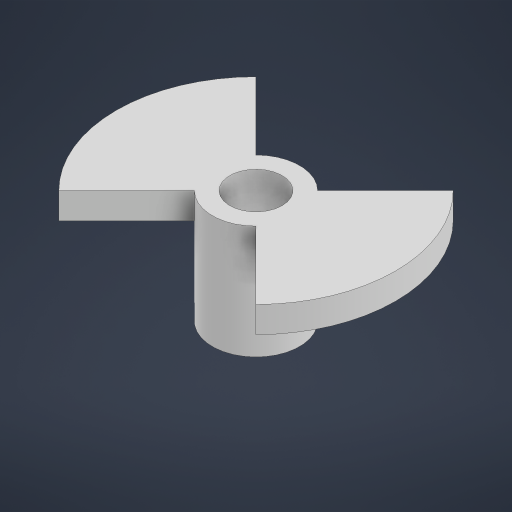
# Autodesk Inventor part: Helice
Saved by Autodesk Inventor 2023.4 (Build 274418000, 418)
## iProperties
Created: 2024-07-01
Part Number: Helice
Material: Generic
Document SubType Name: Modeling
Designer: danni
Density: 1 g/cm^3
Appearance: Default
Author: danni
Autodesk Inventor part; units mm, degrees
ref_plane "YZ Plane" through (0, 0, 0) normal (1, 0, 0) x (0, 1, 0)
ref_plane "XZ Plane" through (0, 0, 0) normal (0, 1, 0) x (-1, 0, 0)
ref_plane "XY Plane" through (0, 0, 0) normal (0, 0, 1) x (1, 0, 0)
sketch "Sketch1" plane through (0, 0, 0) normal (0, 1, 0) x (-1, 0, 0)
  circle A0 centre (0, 0) radius 2.5
  circle A1 centre (0, 0) radius 1.5
  dimension "d1" = 3
  dimension "d2" = 1
  constraints: 2 centre point, 2 coincident
  measures "d1" diameter of A1
  measures "d2" radial gap between concentric circles of A0 A1
extrude "Extrusion1" add sketch "Sketch1" along normal blind 5
sketch "Sketch2" plane through (0, 5, 0) normal (0, 1, 0) x (1, 0, 0)
  circle A0 centre (0, 0) radius 1.5 projected
  circle A1 centre (0, 0) radius 8
  line L0 (-5.6569, -5.6569) -> (5.6569, 5.6569)
  line L1 (-5.6569, 5.6569) -> (5.6569, -5.6569)
  line L2 (-8, 0) -> (8, 0) construction
  circle A2 centre (0, 0) radius 2.5 projected
  point P0 (1.7678, -1.7678)
  point P1 (1.7678, 1.7678)
  point P2 (-1.7678, 1.7678)
  point P3 (-1.7678, -1.7678)
  dimension "d5" = 16
  dimension "d6" = 45
  dimension "d7" = 45
  constraints: 6 end point, 6 point on circle, 3 midpoint, 1 centre point, 1 coincident, 1 horizontal
  measures "d5" diameter of A1
  measures "d6" angle of L2 L1
  measures "d7" angle of L2 L0
extrude "Extrusion2" add sketch "Sketch2" along normal blind 1.5 contours A0 L0 A2 L1 | A0 L1 A2 L0 | L1 A2 L0 A0 | A0 L0 A2 L1 | L0 A1 L1 A2 | A2 L0 A1 L1 picked at (4.6921, -3.9564) picked at (-4.8492, -3.7477)
equation "\"d7\" = d6"
body "Solid1"
